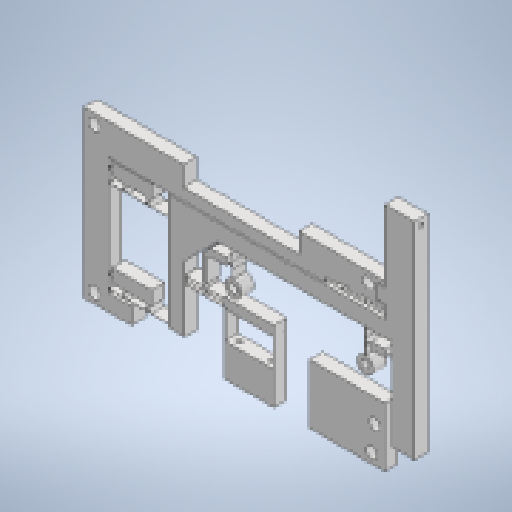
# Autodesk Inventor part: RoueV3PartB
Saved by Autodesk Inventor 2023 (Build 270158000, 158)
## iProperties
Created: 2023-04-29
Part Number: RoueV3PartB
Material: Generic
Document SubType Name: Modeling
Designer: Nathann
Density: 1 g/cm^3
Appearance: Default
Author: Nathann
Autodesk Inventor part; units mm, degrees
ref_plane "YZ Plane" through (0, 0, 0) normal (1, 0, 0) x (0, 1, 0)
ref_plane "XZ Plane" through (0, 0, 0) normal (0, 1, 0) x (-1, 0, 0)
ref_plane "XY Plane" through (0, 0, 0) normal (0, 0, 1) x (1, 0, 0)
sketch "Sketch1" plane through (0, 0, 0) normal (0, 0, 1) x (1, 0, 0)
  line L0 (-50, -25) -> (-50, 25) projected
  line L1 (43, -25) -> (-50, -25) projected
  line L2 (50, 25) -> (50, -10) projected
  line L3 (-50, 25) -> (50, 25) projected
  line L4 (43, -10) -> (50, -10) projected
  line L5 (43, -25) -> (43, -10) projected
  line L6 (43, -10) -> (50, -10)
  line L7 (50, -10) -> (50, -25)
  line L8 (50, -25) -> (43, -25)
  line L9 (43, -25) -> (43, -10)
  point P0 (0, 0)
  constraints: 8 end point, 2 parallel, 1 horizontal, 1 perpendicular
extrude "Extrusion1" add sketch "Sketch1" along normal blind 4
sketch "Sketch2" plane through (0, 0, 4) normal (0, 0, 1) x (1, 0, 0)
  line L0 (50, 25) -> (-50, 25) projected
  line L1 (50, 25) -> (41, 25)
  line L2 (41, 25) -> (41, 45)
  line L3 (41, 45) -> (50, 45)
  line L4 (50, 45) -> (50, 25)
  point P0 (0, 0)
  dimension "d2" = 20
  dimension "d3" = 9
  constraints: 8 end point, 2 parallel, 1 horizontal, 1 perpendicular
  measures "d2" distance between parallel lines of L0 L3
  measures "d3" distance of L2.end L3.end
extrude "Extrusion2" add sketch "Sketch2" against normal blind 4
sketch "Sketch3" plane through (0, 0, 4) normal (0, 0, 1) x (1, 0, 0)
  line L0 (-50, -25) -> (43, -25) projected
  line L1 (50, -25) -> (43, -25)
  line L2 (43, -25) -> (43, -24.5)
  line L3 (43, -24.5) -> (50, -24.5)
  line L4 (50, -24.5) -> (50, -25)
  point P0 (0, 0)
  point P1 (43, -24.75)
  point P2 (43, -25)
  dimension "d6" = 7
  dimension "d7" = 0.5
  constraints: 8 end point, 2 parallel, 1 horizontal, 1 midpoint, 1 perpendicular
  measures "d6" distance from line of point (43, -24.75) L4
  measures "d7" distance between parallel lines of L3 L0
extrude "Extrusion3" cut sketch "Sketch3" against normal blind 4
sketch "Sketch6" plane through (0, 0, 4) normal (0, 0, 1) x (1, 0, 0)
  line L0 (-24.5732, 10) -> (-19.5732, 10)
  line L1 (-19.5732, 10) -> (-19.5732, -20)
  line L2 (-19.5732, -20) -> (-24.5732, -20)
  line L3 (-24.5732, -20) -> (-24.5732, 10)
  line L4 (-50, -25) -> (43, -25) projected
  line L5 (-24.5732, -19) -> (-42.5732, -19)
  line L6 (-42.5732, -19) -> (-42.5732, -18.9)
  line L7 (-42.5732, -18.9) -> (-24.5732, -18.9)
  line L8 (-24.5732, -18.9) -> (-24.5732, -19)
  line L9 (-24.5732, 9) -> (-42.5732, 9)
  line L10 (-42.5732, 9) -> (-42.5732, 8.9)
  line L11 (-42.5732, 8.9) -> (-24.5732, 8.9)
  line L12 (-24.5732, 8.9) -> (-24.5732, 9)
  line L13 (-19.5732, -5.05) -> (-7.5732, -5.05)
  line L14 (-7.5732, -5.05) -> (-7.5732, -4.95)
  line L15 (-7.5732, -4.95) -> (-19.5732, -4.95)
  line L16 (-19.5732, -4.95) -> (-19.5732, -5.05)
  line L17 (-19.5732, 10) -> (43.1, 10)
  line L18 (43.1, 10) -> (43.1, 5)
  line L19 (-19.5732, 5) -> (-19.5732, 10)
  line L20 (43.1, 10) -> (48.1, 10)
  line L21 (48.1, 10) -> (48.1, -24.5)
  line L22 (48.1, -24.5) -> (43.1, -24.5)
  line L23 (43.1, -24.5) -> (43.1, 10)
  line L24 (43, -25) -> (43, -24.5) projected
  line L25 (41, 25) -> (41, 45) projected
  line L26 (50, -10) -> (50, 45) projected
  line L27 (41, 45) -> (50, 45)
  line L28 (50, 45) -> (50, 10)
  line L29 (50, 10) -> (41, 10)
  line L30 (41, 10) -> (41, 45)
  line L31 (43.1, -5.05) -> (25.1, -5.05)
  line L32 (25.1, -5.05) -> (25.1, -4.95)
  line L33 (25.1, -4.95) -> (43.1, -4.95)
  line L34 (43.1, -4.95) -> (43.1, -5.05)
  line L35 (43, -24.5) -> (50, -24.5) projected
  line L36 (-50, 25) -> (-50, -25) projected
  line L37 (-50, -25) -> (43, -25) projected
  line L38 (-50, 25) -> (-42.5732, 25)
  line L39 (-42.5732, 25) -> (-42.5732, -25)
  line L40 (-42.5732, -25) -> (-50, -25)
  line L41 (-50, -25) -> (-50, 25)
  line L42 (25.1, -3.5008) -> (18.1849, -3.5008)
  line L43 (18.1849, -3.5008) -> (18.1849, -25)
  line L44 (18.1849, -25) -> (25.1, -25)
  line L45 (25.1, -25) -> (25.1, -3.5008)
  line L46 (25.1, -25) -> (43, -25)
  line L47 (43, -25) -> (43, -7.05)
  line L48 (43, -7.05) -> (25.1, -7.05)
  line L49 (25.1, -7.05) -> (25.1, -25)
  circle A0 centre (-5, 0) radius 1.2
  circle A1 centre (-5, 0) radius 2.5
  circle A2 centre (35, 0) radius 1.2
  circle A3 centre (35, 0) radius 2.5
  line L50 (-5.05, 10) -> (-4.95, 10)
  line L51 (-4.95, 10) -> (-4.95, 2.3182)
  line L52 (-4.95, 2.3182) -> (-5.05, 2.3182)
  line L53 (-5.05, 2.3182) -> (-5.05, 10)
  line L54 (35.05, 10) -> (34.95, 10)
  line L55 (34.95, 10) -> (34.95, 2.0977)
  line L56 (34.95, 2.0977) -> (35.05, 2.0977)
  line L57 (35.05, 2.0977) -> (35.05, 10)
  line L58 (-42.5732, 25) -> (40.9, 25)
  line L59 (40.9, 17) -> (-42.5732, 17)
  line L60 (-42.5732, 17) -> (-42.5732, 25)
  line L61 (40.9, 23.5) -> (38.9, 23.5)
  line L62 (38.9, 23.5) -> (38.9, 18.5)
  line L63 (38.9, 18.5) -> (40.9, 18.5)
  line L64 (41, 23) -> (39, 23)
  line L65 (39, 23) -> (39, 19)
  line L66 (39, 19) -> (41, 19)
  line L67 (41, 19) -> (41, 23)
  line L68 (40.9, 25) -> (40.9, 23.5)
  line L69 (40.9, 18.5) -> (40.9, 17)
  line L70 (-24.5732, 10) -> (41, 10)
  line L71 (41, 10) -> (41, 15)
  line L72 (41, 15) -> (-24.5732, 15)
  line L73 (-24.5732, 15) -> (-24.5732, 10)
  line L74 (-7.5732, -25) -> (7.4268, -25)
  line L75 (7.4268, -25) -> (7.4268, -15)
  line L76 (7.4268, -15) -> (-7.5732, -15)
  line L77 (-7.5732, -15) -> (-7.5732, -25)
  line L78 (-7.5732, -3.5) -> (7.4268, -3.5)
  line L79 (7.4268, -3.5) -> (7.4268, -6.5)
  line L80 (7.4268, -6.5) -> (-7.5732, -6.5)
  line L81 (-7.5732, -6.5) -> (-7.5732, -3.5)
  line L82 (-7.5732, -6.5) -> (-7.3732, -6.5)
  line L83 (-7.3732, -6.5) -> (-7.3732, -15)
  line L84 (-7.3732, -15) -> (-7.5732, -15)
  line L85 (-7.5732, -15) -> (-7.5732, -6.5)
  line L86 (7.4268, -6.5) -> (7.2268, -6.5)
  line L87 (7.2268, -6.5) -> (7.2268, -15)
  line L88 (7.2268, -15) -> (7.4268, -15)
  line L89 (7.4268, -15) -> (7.4268, -6.5)
  line L90 (-19.5732, -6.05) -> (-7.5732, -6.05)
  line L91 (-7.5732, -6.05) -> (-7.5732, -6.15)
  line L92 (-7.5732, -6.15) -> (-19.5732, -6.15)
  line L93 (-19.5732, -6.15) -> (-19.5732, -6.05)
  line L94 (-7.5732, -3.85) -> (-19.5732, -3.85)
  line L95 (-19.5732, -3.85) -> (-19.5732, -3.95)
  line L96 (-19.5732, -3.95) -> (-7.5732, -3.95)
  line L97 (-7.5732, -3.95) -> (-7.5732, -3.85)
  line L98 (41, 25) -> (-50, 25) projected
  line L99 (40.9, 25) -> (41, 25)
  line L100 (-11.2393, -25) -> (-11.2393, -30) projected
  line L101 (-9.5732, 10) -> (-19.5732, 0)
  line L102 (41, 16.15) -> (23, 16.15)
  line L103 (23, 16.15) -> (23, 16.25)
  line L104 (23, 16.25) -> (41, 16.25)
  line L105 (41, 16.25) -> (41, 16.15)
  line L106 (23, 17) -> (-42.5732, 17)
  line L107 (-42.5732, 17) -> (-42.5732, 15.5)
  line L108 (-42.5732, 15.5) -> (23, 15.5)
  line L109 (23, 15.5) -> (23, 17)
  line L110 (-42.5732, -25) -> (-35.5732, -25)
  line L111 (-35.5732, -25) -> (-35.5732, -20)
  line L112 (-35.5732, -20) -> (-42.5732, -20)
  line L113 (-42.5732, -20) -> (-42.5732, -25)
  line L114 (6.4268, -30) -> (6.4268, -25) projected
  line L115 (-8.5732, -30) -> (-8.5732, -25) projected
  line L116 (6.4268, -30) -> (6.4268, -25) projected
  circle A4 centre (36.05, 5) radius 1
  circle A5 centre (36.05, 7.1) radius 1
  line L117 (37.05, 5) -> (43.1, 5)
  line L118 (37.05, 7.1) -> (43.1, 7.1)
  line L119 (38.6366, 5) -> (40.7366, 5)
  line L120 (40.7366, 5) -> (40.7366, -3.95)
  line L121 (40.7366, -3.95) -> (38.6366, -3.95)
  line L122 (38.6366, -3.95) -> (38.6366, 5)
  circle A6 centre (40.7366, -3.95) radius 1
  circle A7 centre (38.6366, -3.95) radius 1
  circle A8 centre (42.1, 5) radius 1
  circle A9 centre (42.1, 7.1) radius 1
  circle A10 centre (-6.05, 5) radius 1
  circle A11 centre (-6.05, 7.1) radius 1
  line L123 (-6.05, 7.1) -> (-11.7289, 7.1)
  line L124 (-11.7289, 7.1) -> (-11.7289, 5)
  line L125 (-11.7289, 5) -> (-6.05, 5)
  line L126 (-6.05, 5) -> (-6.05, 7.1)
  circle A12 centre (36, 17) radius 0.75
  circle A13 centre (34.4, 17) radius 0.75
  circle A14 centre (29.4, 17) radius 0.75
  circle A15 centre (27.8, 17) radius 0.75
  circle A16 centre (-13.0232, -4.45) radius 0.5
  circle A17 centre (-14.1232, -4.45) radius 0.5
  circle A18 centre (-14.1232, -5.55) radius 0.5
  circle A19 centre (-13.0232, -5.55) radius 0.5
  line L127 (-14.1232, 5) -> (-13.0232, 5)
  line L128 (-13.0232, 5) -> (-13.0232, -3.35)
  line L129 (-13.0232, -3.35) -> (-14.1232, -3.35)
  line L130 (-14.1232, -3.35) -> (-14.1232, 5)
  circle A20 centre (-13.0232, -3.35) radius 0.5
  circle A21 centre (-14.1232, -3.35) radius 0.5
  circle A22 centre (-29.5732, -17.9) radius 1
  circle A23 centre (-31.6732, -17.9) radius 1
  circle A24 centre (-36.6732, -17.9) radius 1
  circle A25 centre (-38.7732, -17.9) radius 1
  line L131 (-29.5732, -16.9) -> (-42.5732, -16.9)
  line L132 (-42.5732, -16.9) -> (-42.5732, -12.8)
  line L133 (-42.5732, -12.8) -> (-29.5732, -12.8)
  line L134 (-29.5732, -12.8) -> (-29.5732, -16.9)
  circle A26 centre (-42.5732, -15.9) radius 1
  circle A27 centre (-42.5732, -13.8) radius 1
  circle A28 centre (-29.5732, 10) radius 1
  circle A29 centre (-31.6732, 10) radius 1
  circle A30 centre (-36.6732, 10) radius 1
  circle A31 centre (-38.7732, 10) radius 1
  line L135 (-29.5732, 11) -> (-42.5732, 11)
  line L136 (-42.5732, 11) -> (-42.5732, 15.1)
  line L137 (-42.5732, 15.1) -> (-29.5732, 15.1)
  line L138 (-29.5732, 15.1) -> (-29.5732, 11)
  circle A32 centre (-42.5732, 12) radius 1
  circle A33 centre (-42.5732, 14.1) radius 1
  line L139 (-41.5732, 15.1) -> (-41.5732, 14.1)
  line L140 (-41.5732, 12) -> (-41.5732, 11)
  line L141 (-41.5732, -15.9) -> (-41.5732, -16.9)
  line L142 (-41.5732, -13.8) -> (-41.5732, -12.8)
  line L143 (-11.7289, 7.1) -> (-14.1232, 5)
  line L144 (-11.7289, 5) -> (-13.0232, 3.8648)
  point P0 (0, 0)
  point P1 (-7.5732, -5)
  point P2 (43.1, -5)
  point P3 (-5, 10)
  point P4 (35, 10)
  point P5 (-42.5732, 8.95)
  point P6 (-42.5732, -18.95)
  point P7 (7.2268, -6.5)
  point P8 (-7.3732, -6.5)
  point P9 (-42.5732, -25)
  point P10 (-7.5732, -25)
  point P11 (43.1, -4.95)
  point P12 (35.05, 10)
  point P13 (35.05, 2.4995)
  point P14 (34.95, 2.4995)
  point P15 (34.95, 10)
  point P16 (-4.95, 10)
  point P17 (-4.95, 2.4995)
  point P18 (-5.05, 2.4995)
  point P19 (-5.05, 10)
  point P20 (7.4268, -25)
  point P21 (25.1, -7.05)
  point P22 (-7.5732, -4.95)
  point P23 (-42.5732, 8.9)
  point P24 (-42.5732, -18.9)
  point P25 (-24.5732, 8.9)
  point P26 (-42.5732, 17)
  point P27 (25.1, -5)
  point P28 (25.1, -5.05)
  point P29 (25.1, -4.95)
  point P30 (-9.5732, 10)
  point P31 (23, 16.2)
  point P32 (-42.5732, 16.25)
  point P33 (-35.5732, -25)
  point P34 (-31.6732, 11)
  point P35 (-36.6732, 11)
  point P36 (-36.6732, 9)
  point P37 (-31.6732, 9)
  point P38 (-42.5732, 13)
  point P39 (-38.7732, 11)
  point P40 (-38.7732, 9)
  point P41 (-29.5732, 9)
  point P42 (-42.5732, 13.1)
  point P43 (36, 16.25)
  point P44 (36.75, 17)
  point P45 (29.4, 16.25)
  point P46 (34.4, 16.25)
  point P47 (33.65, 17)
  point P48 (30.15, 17)
  point P49 (27.05, 17)
  point P50 (27.8, 16.25)
  point P51 (35.05, 7.1)
  point P52 (41.1, 7.1)
  point P53 (-5.05, 7.1)
  point P54 (-12.4732, 7.1)
  point P55 (-7.05, 7.1)
  point P56 (-14.1232, -3.85)
  point P57 (-14.1232, -2.85)
  point P58 (-14.1862, 5)
  point P59 (41.1, 5)
  point P60 (35.05, 5)
  point P61 (-5.05, 5)
  point P62 (-7.05, 5)
  point P63 (-13.0232, -2.85)
  point P64 (-13.0232, -3.85)
  point P65 (-31.6732, -16.9)
  point P66 (-36.6732, -16.9)
  point P67 (-36.6732, -18.9)
  point P68 (-31.6732, -18.9)
  point P69 (-42.5732, -14.9)
  point P70 (-38.7732, -16.9)
  point P71 (-38.7732, -18.9)
  point P72 (-42.5732, -14.8)
  point P73 (-29.5732, -18.9)
  point P74 (-13.0232, -4.95)
  point P75 (-13.0232, -3.95)
  point P76 (-14.1232, -3.95)
  point P77 (-14.1232, -4.95)
  point P78 (-14.1232, -5.05)
  point P79 (-14.1232, -6.05)
  point P80 (-13.0232, -6.05)
  point P81 (-13.0232, -5.05)
  point P82 (-6.05, 6.1)
  point P83 (-13.6232, -3.35)
  point P84 (-19.5732, -3.85)
  point P85 (-6.05, 6)
  point P86 (-13.5232, -3.35)
  dimension "d142" = 2
  dimension "d143" = 2
  dimension "d168" = 2
  dimension "d179" = 2
  dimension "d27" = 5
  dimension "d28" = 30
  dimension "d29" = 18
  dimension "d30" = 0.1
  dimension "d31" = 1
  dimension "d32" = 0.1
  dimension "d33" = 1
  dimension "d34" = 15
  dimension "d35" = 0.1
  dimension "d37" = 5
  dimension "d39" = 5
  dimension "d40" = 0.1
  dimension "d41" = 0.1
  dimension "d43" = 0
  dimension "d44" = 15
  dimension "d45" = 18
  dimension "d46" = 2
  dimension "d47" = 0.1
  dimension "d48" = 40
  dimension "d49" = 2.4
  dimension "d50" = 2.4
  dimension "d51" = 5
  dimension "d52" = 5
  dimension "d53" = 0.1
  dimension "d54" = 0.05
  dimension "d55" = 0.05
  dimension "d56" = 0.1
  dimension "d57" = 8
  dimension "d59" = 2
  dimension "d60" = 1.5
  dimension "d61" = 5
  dimension "d62" = 0.5
  dimension "d63" = 0.5
  dimension "d64" = 0.1
  dimension "d65" = 0.1
  dimension "d66" = 5
  dimension "d67" = 0
  dimension "d68" = 0
  dimension "d69" = 15
  dimension "d70" = 10
  dimension "d71" = 15
  dimension "d72" = 0
  dimension "d73" = 1.5
  dimension "d74" = 1.5
  dimension "d75" = 0.2
  dimension "d76" = 0.2
  dimension "d79" = 1
  dimension "d80" = 0.1
  dimension "d81" = 0.1
  dimension "d82" = 1
  dimension "d87" = 15
  dimension "d88" = 10
  dimension "d89" = 10
  dimension "d90" = 10
  dimension "d91" = 10
  dimension "d92" = 0.1
  dimension "d93" = 0.75
  dimension "d94" = 2
  dimension "d95" = 1.5
  dimension "d97" = 18
  dimension "d130" = 0.1
  dimension "d131" = 7
  dimension "d132" = 5
  dimension "d135" = 12
  constraints: 264 end point, 61 parallel, 48 point on line, 36 horizontal, 32 perpendicular, 28 centre point, 19 tangent, 10 midpoint, 8 point on circle, 4 vertical, 3 coincident, 26 other
  measures "d27" distance between parallel lines of L4 L2
  measures "d28" distance of L2.end L0.start
  measures "d29" distance of L5.start L5.end
  measures "d30" distance of L5.end L6.end
  measures "d31" distance between parallel lines of L2 L5
  measures "d32" distance between parallel lines of L11 L9
  measures "d33" distance between parallel lines of L0 L9
  measures "d34" distance from line of L0 point (-7.573, -5)
  measures "d35" distance between parallel lines of L15 L13
  measures "d37" distance of L0.start L0.end
  measures "d39" distance of L21.end L22.end
  measures "d40" distance between parallel lines of L23 L24
  measures "d41" distance between parallel lines of L33 L31
  measures "d43" distance between parallel lines of L35 L22
  measures "d44" distance from line of L17 point (43.1, -5)
  measures "d45" distance of L31.start L31.end
  measures "d46" distance between parallel lines of L48 L31
  measures "d47" distance between parallel lines of L23 L47
  measures "d48" distance of A2.centre A0.centre
  measures "d49" diameter of A0
  measures "d50" diameter of A2
  measures "d51" diameter of A3
  measures "d52" diameter of A1
  measures "d53" distance between parallel lines of L57 L55
  measures "d54" distance from line of L55 A2.centre
  measures "d55" distance from line of L51 A0.centre
  measures "d56" distance between parallel lines of L51 L53
  measures "d57" distance between parallel lines of L58 L59
  measures "d59" distance of L61.start L61.end
  measures "d60" distance between parallel lines of L58 L61
  measures "d61" distance of L61.end L62.end
  measures "d62" distance between parallel lines of L61 L64
  measures "d63" distance between parallel lines of L63 L66
  measures "d64" distance between parallel lines of L30 L68
  measures "d65" distance between parallel lines of L30 L69
  measures "d66" distance between parallel lines of L70 L72
  measures "d67" distance from line of L17 point (-5, 10)
  measures "d68" distance from line of L70 point (35, 10)
  measures "d69" distance of L75.end L76.end
  measures "d70" distance of L76.end L74.start
  measures "d71" distance of L78.start L78.end
  measures "d72" distance between parallel lines of L75 L79
  measures "d73" distance from line of L78 point (-7.573, -5)
  measures "d74" distance from line of L80 point (-7.573, -5)
  measures "d75" distance between parallel lines of L83 L85
  measures "d76" distance between parallel lines of L89 L87
  measures "d79" distance between parallel lines of L15 L96
  measures "d80" distance between parallel lines of L96 L94
  measures "d81" distance between parallel lines of L92 L90
  measures "d82" distance between parallel lines of L13 L90
  measures "d87" distance from line of L26 A2.centre
  measures "d88" distance from line of L17 A0.centre
  measures "d89" distance from line of L70 A3.centre
  measures "d90" distance of L0.end L101.start
  measures "d91" distance of L0.end L101.end
  measures "d92" distance between parallel lines of L104 L102
  measures "d93" distance between parallel lines of L59 L104
  measures "d94" distance between parallel lines of L59 L72
  measures "d95" distance between parallel lines of L59 L108
  measures "d97" distance of L102.start L102.end
  measures "d130" distance between parallel lines of L65 L62
  measures "d131" distance of L111.end L112.end
  measures "d132" distance of L110.end L111.end
  measures "d135" distance between parallel lines of L1 L85
extrude "Extrusion4" cut sketch "Sketch6" against normal blind 4 contours L3 L9 A28 L138 L137 L39 L108 L109 L102 L30 L72 L73 | L17 L53 A11 L123 L143 L130 A21 L94 L1 L101 | L3 L7 A22 L134 L133 L39 L11 | A28 | L9 A30 L135 A29 | A29 | L17 L18 A9 L118 A5 L57 | L17 L55 A3 L57 A4 L117 L122 A7 L33 L45 L42 L43 L4 L75 L89 L79 L78 L81 L94 A20 L128 L144 L125 A10 L53 A1 L51 | A11 L126 L123 | L3 L2 L1 L92 L81 L85 L77 L4 L111 L112 L39 L5 | A22 | L39 L135 A31 L9 | A27 L39 | L133 L142 A27 | A30 | L104 A12 L59 L69 L63 L62 L61 L68 L98 L30 L64 L65 L66 | L96 A17 L15 L1 | A21 L130 L129 | L51 L52 L53 A1 | A10 L125 L126 | L123 L126 A11 | L7 A24 L131 A23 | A23 | A31 | A32 L140 L135 | L39 A32 | L139 A33 L137 | A5 | A9 L118 | L118 A9 | A12 L59 | L109 L59 A15 L104 | A17 | A20 L129 L128 | A21 L129 L130 | L126 L125 A10 | L39 L131 A25 L7 | A24 | A26 L39 | A33 L39 | A4 | A8 L117 | L117 A8 | L23 L33 A6 L120 L117 A8 | L104 A14 L59 A13 | A13 L59 | A12 L59 | A15 L59 | L13 A18 L90 L1 | L96 L81 L15 A16 | A16 | A20 L128 L129 | A25 | A26 L141 L131 | L23 L31 L32 L33 | L35 L47 L48 L45 L31 L23 | A14 L59 | A13 L59 | A15 L59 | A18 | L117 L120 A6 L121 A7 L122 | L33 A7 L121 A6 | A6 L121 L120 | A14 L59 | L13 L81 L90 A19 | A19 | A7 L121 L122 | L122 L121 A7 | A6 L120 L121 | L80 L87 L76 L83 | A0 | A2 picked at (-42.2399, -13.8) picked at (-4.9944, 2.3788) picked at (-42.2399, 12) picked at (-42.2399, -15.9) picked at (-42.2399, 14.1)
sketch "Sketch7" plane through (0, 0, 4) normal (0, 0, 1) x (1, 0, 0)
  line L0 (43, -24.5) -> (50, -24.5) projected
  line L1 (43.1, -24.5) -> (43.1, 5) projected
  line L2 (50, -24.5) -> (43.1, -24.5)
  line L3 (43.1, -24.5) -> (43.1, -17.5)
  line L4 (43.1, -17.5) -> (50, -17.5)
  line L5 (50, -17.5) -> (50, -24.5)
  line L6 (43, -24.5) -> (43, -25) projected
  line L7 (43, -25) -> (41, -25)
  line L8 (41, -25) -> (41, -5)
  line L9 (41, -5) -> (43, -5)
  line L10 (43, -5) -> (43, -25)
  point P0 (0, 0)
  point P1 (43.1, 10)
  point P2 (43, -7.05)
  point P3 (43, -10)
  point P4 (43, -7.05)
  point P5 (43.1, -4.95)
  dimension "d98" = 7
  dimension "d105" = 2
  dimension "d106" = 6.9
  dimension "d107" = 20
  constraints: 16 end point, 4 parallel, 2 horizontal, 2 perpendicular, 1 point on line
  measures "d98" distance between parallel lines of L0 L4
  measures "d105" distance of L6.end L7.end
  measures "d106" distance of L1.start L0.end
  measures "d107" distance of L7.end L8.end
extrude "Extrusion5" cut sketch "Sketch7" against normal blind 4
sketch "Sketch9" plane through (0, 0, 4) normal (0, 0, 1) x (1, 0, 0)
  line L0 (41, 25) -> (-50, 25) projected
  line L1 (15, 25) -> (-20, 25)
  line L2 (-20, 25) -> (-20, 19)
  line L3 (-20, 19) -> (15, 19)
  line L4 (15, 19) -> (15, 25)
  line L5 (50, -17.5) -> (50, 45) projected
  line L6 (-50, 25) -> (-50, -25) projected
  point P0 (0, 0)
  point P1 (40.9, 25)
  point P2 (-20, 25)
  dimension "d108" = 35
  dimension "d110" = 6
  dimension "d121" = 30
  constraints: 8 end point, 2 parallel, 1 horizontal, 1 perpendicular, 1 point on line
  measures "d108" distance of L2.end L3.end
  measures "d110" distance of L1.end L2.end
  measures "d121" distance between parallel lines of L6 L2
extrude "Extrusion7" cut sketch "Sketch9" against normal blind 4
sketch "Sketch10" plane through (-7.5732, -25, 0) normal (0, -1, 0) x (1, 0, 0)
  circle A0 centre (2.5, 2) radius 0.8
  circle A1 centre (12.5, 2) radius 0.8
  line L0 (-42.4268, 4) -> (15, 4) projected
  line L1 (0, 4) -> (0, 0) projected
  point P0 (7.5732, 0)
  point P1 (50.5732, 4)
  point P2 (25.7581, 4)
  dimension "d113" = 2
  dimension "d114" = 2
  dimension "d115" = 10
  dimension "d116" = 2.5
  dimension "d117" = 1.6
  dimension "d118" = 1.6
  constraints: 2 centre point
  measures "d113" distance from line of L0 A0.centre
  measures "d114" distance from line of L0 A1.centre
  measures "d115" distance of A0.centre A1.centre
  measures "d116" distance from line of L1 A0.centre
  measures "d117" diameter of A0
  measures "d118" diameter of A1
extrude "Extrusion8" cut sketch "Sketch10" against normal blind 10
sketch "Sketch11" plane through (0, 0, 4) normal (0, 0, 1) x (1, 0, 0)
  circle A0 centre (28, -22) radius 1.7 projected
  circle A1 centre (38, -14) radius 1.7 projected
  circle A2 centre (28.5, 22.5) radius 1.7 projected
  circle A3 centre (-47, 22) radius 1.7 projected
  circle A4 centre (-47, -22) radius 1.7 projected
  line L0 (41, -25) -> (41, -7.05) projected
  circle A5 centre (37, -22) radius 1.7
  line L1 (-50, -25) -> (-35.5732, -25) projected
  circle A6 centre (36, 22) radius 1.7 projected
  point P0 (0, 0)
  point P1 (18.1849, -25)
  point P2 (41, -5)
  dimension "d124" = 13
  dimension "d125" = 3
  dimension "d126" = 3
  dimension "d127" = 4
  dimension "d128" = 3.4
  dimension "d129" = 3.4
  constraints: 1 centre point
  measures "d124" distance from line of L0 A0.centre
  measures "d125" distance from line of L1 A0.centre
  measures "d126" distance from line of L1 A5.centre
  measures "d127" distance from line of L0 A5.centre
  measures "d128" diameter of A0
  measures "d129" diameter of A5
extrude "Extrusion9" cut sketch "Sketch11" against normal blind 10 contours A1 | A3 | A4 | A5 | A6
sketch "Sketch12" plane through (0, 0, 4) normal (0, 0, 1) x (1, 0, 0)
  line L0 (25.1, -7.05) -> (25.1, -3.5008) projected
  line L1 (25.1, -7.05) -> (18.1849, -7.05)
  line L2 (18.1849, -7.05) -> (18.1849, -3.5008)
  line L3 (18.1849, -3.5008) -> (25.1, -3.5008)
  line L4 (25.1, -3.5008) -> (25.1, -7.05)
  point P0 (0, 0)
  constraints: 8 end point, 2 parallel, 1 horizontal, 1 perpendicular
extrude "Extrusion10" cut sketch "Sketch12" against normal blind 8
sketch "Sketch13" plane through (50, 45, 4) normal (1, 0, 0) x (0, 0, -1)
  circle A0 centre (2, -2) radius 0.255
  line L0 (0, 0) -> (4, 0) projected
  line L1 (0, -62.5) -> (0, 0) projected
  point P0 (4, -45)
  dimension "d195" = 2
  dimension "d196" = 2
  dimension "d197" = 0.51
  constraints: 1 centre point
  measures "d195" distance from line of L0 A0.centre
  measures "d196" distance from line of L1 A0.centre
  measures "d197" diameter of A0
extrude "Extrusion11" cut sketch "Sketch13" against normal blind 20
equation "\"d52\" = d51"
equation "\"d54\" = 0.5 * d53"
equation "\"d55\" = 0.5 * d56"
equation "\"d74\" = d73"
equation "\"d82\" = d79"
equation "\"bladeThicknessTablePushing\" = 0.1"
equation "\"bladeThicknessTable\" = 0.1"
equation "\"bladeThicknessForceConverter\" = 0.2"
equation "\"bladeThicknessWheelAnchor\" = 0.1"
equation "\"safetyPlay\" = 0.1"
equation "\"OffsetMotorSpring\" = -1"
equation "\"BladeThicknessRCC\" = 0.1"
equation "\"bladeThicknessZeroConverter\" = 0.1"
equation "\"rangeXProbeMin\" = -0.6"
equation "\"thicknessWheelPlate\" = 8"
equation "\"rangeXProbeMax\" = 0.6"
equation "\"BladeLengthRCC\" = 18"
equation "\"bladeLengthTable\" = 18"
equation "\"bladeLengthWheelAnchor\" = 7.5"
equation "\"RCCdeadCenter\" = 5"
equation "\"bladeLengthZeroConverter\" = 11.98"
equation "\"bladeLengthTablePushing\" = 12"
equation "\"bladeLengthForceConverter\" = 12.125"
equation "\"thicknessConverterPlate\" = 4"
body "Solid1"
